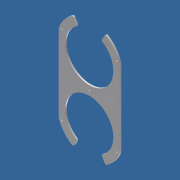
# Autodesk Inventor part: J001393
Saved by Autodesk Inventor 2012 SP2 (Build 160219200, 219)
## iProperties
Created: 2012-04-07
Part Number: J001393
Material: ALUMINUM, 6061-T651
Document SubType Name: Modeling
Designer: Igor
Density: 2.7 g/cm^3
Mass: 766.965 g
Surface Area: 1041.38 cm^2
Volume: 284.061 cm^3
Project: P-51601
Description: TOP PLATE
Vendor: HHMI: JFRC - ID&F
SPECIAL FINISH: ANODIZE PER MIL-A-8625F, TYPE II, CLASS 2 (BLACK)
ALTERED ITEM PART NUMBER: N/A
ALTERED ITEM VENDOR: N/A
DESIGN DEPARTMENT: HHMI: JFRC - ID&F
LAB/DEPT: GONEN (LAB)
REQUESTING SCIENTIST: GONEN, TAMIR
SURFACE ROUGHNESS: 32 Ra
ALTERED ITEM DESCRIPTION: N/A
Author: Igor
Revision Number: -
Autodesk Inventor part; units mm, degrees
ref_plane "YZ Plane" through (0, 0, 0) normal (1, 0, 0) x (0, 1, 0)
ref_plane "XZ Plane" through (0, 0, 0) normal (0, 1, 0) x (-1, 0, 0)
ref_plane "XY Plane" through (0, 0, 0) normal (0, 0, 1) x (1, 0, 0)
sketch "Sketch1" plane through (0, 0, 0) normal (0, 0, 1) x (1, 0, 0)
  arc A0 (50.165, -86.8883) -> (-50.165, -86.8883) centre (0, 0) ccw
  line L0 (0, 123.825) -> (0, 0) construction
  line L1 (-168.8677, 119.38) -> (168.8677, 119.38) construction
  line L2 (127, 119.38) -> (127, -44.6491)
  line L3 (0, 0) -> (67.31, -116.5843) construction
  line L4 (50.165, -86.8883) -> (67.31, -116.5843)
  line L5 (-127, 119.38) -> (-127, -44.6491)
  line L6 (0, 0) -> (-67.31, -116.5843) construction
  line L7 (-50.165, -86.8883) -> (-67.31, -116.5843)
  arc A1 (-50.165, 325.6483) -> (50.165, 325.6483) centre (0, 238.76) ccw
  line L8 (127, 119.38) -> (127, 283.4091)
  line L9 (50.165, 325.6483) -> (67.31, 355.3443)
  line L10 (-127, 119.38) -> (-127, 283.4091)
  line L11 (-50.165, 325.6483) -> (-67.31, 355.3443)
  arc A2 (127, 283.4091) -> (67.31, 355.3443) centre (0, 238.76) ccw
  arc A3 (-67.31, 355.3443) -> (-127, 283.4091) centre (0, 238.76) ccw
  arc A4 (-127, -44.6491) -> (-67.31, -116.5843) centre (0, 0) ccw
  arc A5 (67.31, -116.5843) -> (127, -44.6491) centre (0, 0) ccw
  point P0 (114.3, -45.72)
  point P1 (0, 119.38)
  point P2 (-114.3, -45.72)
  point P3 (114.3, 284.48)
  point P4 (-114.3, 284.48)
  dimension "d1" = 200.66
  dimension "d18" = 119.38
  dimension "d19" = 165.1
  dimension "d20" = 114.3
  dimension "d25" = 127
  dimension "d26" = 150
  dimension "d34" = 134.62
  constraints: 24 end point, 14 symmetric about line, 12 point on circle, 6 centre point, 2 coincident, 2 collinear, 2 vertical, 1 horizontal, 1 midpoint, 1 point on line, 1 other
  measures "d1" diameter of A0
  measures "d18" distance from line of point (0, 0) L1
  measures "d19" distance from line of point (114.3, -45.72) L1
  measures "d20" distance from line of point (114.3, -45.72) L0
  measures "d25" distance between parallel lines of L2 L0
  measures "d26" angle of L3 L0
  measures "d34" radius of A5
extrude "Extrusion1" add sketch "Sketch1" along normal blind 6.35
hole "Hole2" at (114.3, -45.72, 0) at (0, 119.38, 0) at (-114.3, -45.72, 0) at (114.3, 284.48, 0) at (-114.3, 284.48, 0) direction (0, 0, 1) diameter 6.7564 end through all clearance for "Flat Head Machine Screw (82)" size "1/4" standard "Ansi Unified Screw Threads"
fillet "Fillet1" radius 6.35 8 edges at (50.165, -86.8883, 3.175) (-50.165, -86.8883, 3.175) (67.31, 355.3443, 3.175) (-67.31, 355.3443, 3.175) (50.165, 325.6483, 3.175) (-50.165, 325.6483, 3.175) (67.31, -116.5843, 3.175) (-67.31, -116.5843, 3.175)
body "Solid1"
